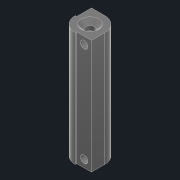
# Autodesk Inventor part: base6
Saved by Autodesk Inventor 2022 (Build 260153000, 153)
## iProperties
Created: 2021-07-22
Part Number: base6
Material: ABS プラスチック
Document SubType Name: Modeling
Designer: yuta0
Density: 1.06 g/cm^3
Appearance: 滑らか - 黒
Mass: 26.982 g
Surface Area: 66.0467 cm^2
Volume: 25.4547 cm^3
購入先: 印刷
在庫数: 0.0
Author: yuta0
Autodesk Inventor part; units mm, degrees
ref_plane "YZ Plane" through (0, 0, 0) normal (1, 0, 0) x (0, 1, 0)
ref_plane "XZ Plane" through (0, 0, 0) normal (0, 1, 0) x (-1, 0, 0)
ref_plane "XY Plane" through (0, 0, 0) normal (0, 0, 1) x (1, 0, 0)
sketch "スケッチ1" plane through (0, 0, 0) normal (0, 1, 0) x (-1, 0, 0)
  circle A0 centre (0, 0) radius 10
  line L0 (0, 10) -> (-10, 10)
  line L1 (-10, 10) -> (-10, -10)
  line L2 (-10, -10) -> (10, -10)
  line L3 (10, -10) -> (10, 0)
  dimension "d0" = 20
  dimension "d1" = 10
  dimension "d2" = 10
  constraints: 8 end point, 3 perpendicular, 2 point on circle, 2 tangent, 1 centre point, 1 coincident, 1 horizontal
  measures "d0" diameter of A0
  measures "d1" distance of L2.end L3.end
  measures "d2" distance of L0.start L0.end
extrude "押し出し1" add sketch "スケッチ1" along normal blind 77
sketch "スケッチ2" plane through (0, 0, 10) normal (0, 0, 1) x (1, 0, 0)
  line L0 (0, 0) -> (0, 77) projected
  line L1 (0, 77) -> (10, 77) projected
  line L2 (10, 77) -> (10, 0) projected
  line L3 (10, 0) -> (0, 0) projected
extrude "押し出し2" cut sketch "スケッチ2" against normal blind 1
sketch "スケッチ3" plane through (-10, 0, -10) normal (-1, 0, 0) x (0, 0, 1)
  line L0 (0, 77) -> (10, 77) projected
  line L1 (10, 0) -> (10, 77) projected
  line L2 (10, 0) -> (0, 0) projected
  line L3 (0, 0) -> (0, 77) projected
extrude "押し出し3" cut sketch "スケッチ3" against normal blind 1
sketch "スケッチ4" plane through (0, 0, 9) normal (0, 0, 1) x (1, 0, 0)
  line L0 (0, 77) -> (10, 77) projected
  line L1 (10, 77) -> (10, 0) projected
  line L2 (10, 0) -> (0, 0) projected
  point P0 (5, 72)
  point P1 (5, 5)
  dimension "d9" = 5
  dimension "d10" = 5
  dimension "d11" = 5
  constraints: 1 vertical alignment
  measures "d9" distance from line of L0 point (5, 72)
  measures "d10" distance from line of point (5, 72) L1
  measures "d11" distance from line of L2 point (5, 5)
hole "穴1" at (5, 72, 9) at (5, 5, 9) direction (0, 0, -1) diameter 5 depth 6 tip angle 118
sketch "スケッチ5" plane through (0, 0, 0) normal (0, 1, 0) x (1, 0, 0)
  point P0 (0, 0)
hole "穴2" at (0, 0, 0) direction (0, 1, 0) diameter 5 depth 6 tip angle 118
sketch "スケッチ6" plane through (-9, 0, -10) normal (-1, 0, 0) x (0, 0, 1)
  line L0 (0, 0) -> (0, 77) projected
  line L1 (0, 77) -> (10, 77) projected
  line L2 (10, 0) -> (0, 0) projected
  point P0 (5, 72)
  point P1 (5, 5)
  dimension "d26" = 5
  dimension "d27" = 5
  dimension "d28" = 5
  dimension "d29" = 5
  measures "d26" distance from line of L0 point (5, 72)
  measures "d27" distance from line of L1 point (5, 72)
  measures "d28" distance from line of L2 point (5, 5)
  measures "d29" distance from line of L0 point (5, 5)
hole "穴3" at (-9, 72, -5) at (-9, 5, -5) direction (1, 0, 0) diameter 5 depth 6 tip angle 118
sketch "スケッチ7" plane through (0, 77, 0) normal (0, 1, 0) x (1, 0, 0)
  circle A0 centre (0, 0) radius 3.05
  dimension "d37" = 6.1
  constraints: 1 centre point, 1 coincident
  measures "d37" diameter of A0
extrude "押し出し4" cut sketch "スケッチ7" against normal blind 6
chamfer "面取り1" distance 3 angle 45 1 edges at (-3.05, 77, 0)
fillet "フィレット1" radius 10 1 edges at (10, 38.5, -10)
equation "\"d11\" = d9"
